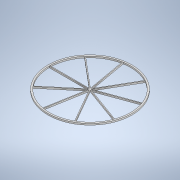
# Autodesk Inventor part: Деталь2
Saved by Autodesk Inventor 2022 (Build 260153000, 153)
## iProperties
Created: 2023-03-14
Part Number: Деталь2
Material: Типовые
Document SubType Name: Modeling
Designer: lrnto01
Density: 1 g/cm^3
Appearance: По умолчанию
Author: lrnto01
Autodesk Inventor part; units mm, degrees
ref_plane "YZ Plane" through (0, 0, 0) normal (1, 0, 0) x (0, 1, 0)
ref_plane "XZ Plane" through (0, 0, 0) normal (0, 1, 0) x (-1, 0, 0)
ref_plane "XY Plane" through (0, 0, 0) normal (0, 0, 1) x (1, 0, 0)
sketch "Эскиз1" plane through (0, 0, 0) normal (0, 1, 0) x (-1, 0, 0)
  circle A0 centre (0, 0) radius 55
  line L0 (0, 0) -> (0, -0.5)
  line L1 (0, 0) -> (0, 0.5)
  line L2 (1.3737, 0.5) -> (52.9976, 0.5)
  arc A1 (52.9976, 0.5) -> (40.9199, 33.6832) centre (0, 0) ccw
  arc A2 (40.2772, 34.4492) -> (9.6953, 52.1057) centre (0, 0) ccw
  arc A3 (8.7105, 52.2793) -> (-26.0658, 46.1473) centre (0, 0) ccw
  arc A4 (-26.9318, 45.6473) -> (-49.6305, 18.5961) centre (0, 0) ccw
  arc A5 (-49.9725, 17.6564) -> (-49.9725, -17.6564) centre (0, 0) ccw
  arc A6 (-49.6305, -18.5961) -> (-26.9318, -45.6473) centre (0, 0) ccw
  arc A7 (-26.0658, -46.1473) -> (8.7105, -52.2793) centre (0, 0) ccw
  arc A8 (9.6953, -52.1057) -> (40.2772, -34.4492) centre (0, 0) ccw
  arc A9 (40.9199, -33.6832) -> (52.9976, -0.5) centre (0, 0) ccw
  line L3 (-1.1199, 0.9397) -> (-49.6305, 18.5961)
  line L4 (-1.1199, 0.9397) -> (-26.9318, 45.6473)
  line L5 (-1.4619, 0) -> (-49.9725, -17.6564)
  line L6 (-1.4619, 0) -> (-49.9725, 17.6564)
  line L7 (-1.1199, -0.9397) -> (-26.9318, -45.6473)
  line L8 (0.0882, -0.5) -> (0, -0.5321)
  line L9 (-1.1199, -0.9397) -> (-49.6305, -18.5961)
  line L10 (-0.2539, -1.4397) -> (8.7105, -52.2793)
  line L11 (0.731, -1.266) -> (40.2772, -34.4492)
  line L12 (0.3889, -0.3264) -> (0.342, -0.4076)
  line L13 (-0.2539, -1.4397) -> (-26.0658, -46.1473)
  line L14 (0.731, -1.266) -> (9.6953, -52.1057)
  line L15 (0.3214, -0.383) -> (0.3889, -0.3264)
  line L16 (0.7779, 0) -> (40.9199, 33.6832)
  line L17 (0.7779, 0) -> (40.9199, -33.6832)
  line L18 (0.731, 1.266) -> (9.6953, 52.1057)
  line L19 (0.731, 1.266) -> (40.2772, 34.4492)
  line L20 (-0.2539, 1.4397) -> (-26.0658, 46.1473)
  line L21 (-0.2539, 1.4397) -> (8.7105, 52.2793)
  line L22 (0, -0.5) -> (0.0882, -0.5)
  line L23 (1.3737, -0.5) -> (52.9976, -0.5)
  dimension "d0" = 110
  dimension "d2" = 0.5
  dimension "d3" = 0.5
  constraints: 48 end point, 18 point on circle, 10 centre point, 4 point on line, 3 perpendicular, 2 coincident, 1 vertical
  measures "d0" diameter of A0
  measures "d2" distance of L0.start L0.end
  measures "d3" distance of L0.start L1.end
extrude "Выдавливание1" add sketch "Эскиз1" along normal blind 2
